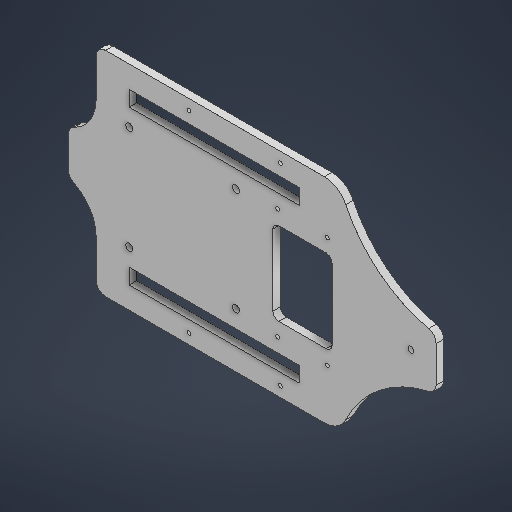
# Autodesk Inventor part: platform_deck
Saved by Autodesk Inventor 2026.1 (Build 301233020, 233B)
## iProperties
Created: 2026-01-28
Part Number: platform_deck
Material: Genérico
Document SubType Name: Modeling
Designer: i5
Density: 1 g/cm^3
Appearance: Valor por defecto
Author: i5
Autodesk Inventor part; units mm, degrees
ref_plane "YZ Plane" through (0, 0, 0) normal (1, 0, 0) x (0, 1, 0)
ref_plane "XZ Plane" through (0, 0, 0) normal (0, 1, 0) x (-1, 0, 0)
ref_plane "XY Plane" through (0, 0, 0) normal (0, 0, 1) x (1, 0, 0)
sketch "Boceto1" plane through (0, 0, 0) normal (0, 0, 1) x (1, 0, 0)
  line L0 (110.3805, 161.5) -> (194.7805, 161.5)
  line L1 (110.3805, 161.5) -> (194.7805, 161.5)
  line L2 (194.7805, 161.5) -> (194.7805, 148.5)
  line L3 (194.7805, 148.5) -> (110.3805, 148.5)
  line L4 (110.3805, 180) -> (216.0805, 180)
  line L5 (310.3805, 90) -> (310.3805, 105.2)
  arc A0 (310.3805, 105.2) -> (304.1178, 113.0091) centre (302.3805, 105.2) ccw
  arc A1 (234.1183, 168.6393) -> (216.0805, 180) centre (216.0805, 160) ccw
  arc A2 (234.1183, 168.6393) -> (304.1178, 113.0091) centre (326.3176, 212.7984) ccw
  line L6 (172.5805, 90) -> (172.5805, 120)
  line L7 (222.5805, 120) -> (222.5805, 90)
  circle A3 centre (289.0805, 90) radius 2.5
  circle A4 centre (141.4805, 133.75) radius 3
  line L8 (177.5805, 125) -> (197.5805, 125)
  arc A5 (177.5805, 125) -> (172.5805, 120) centre (177.5805, 120) ccw
  circle A6 centre (176.5805, 136.75) radius 1.65
  circle A7 centre (218.5805, 136.75) radius 1.65
  circle A8 centre (178.8805, 171.35) radius 1.65
  line L9 (197.5805, 125) -> (217.5805, 125)
  arc A9 (222.5805, 120) -> (217.5805, 125) centre (217.5805, 120) ccw
  line L10 (110.3805, 18.5) -> (194.7805, 18.5)
  line L11 (110.3805, 18.5) -> (194.7805, 18.5)
  line L12 (194.7805, 18.5) -> (194.7805, 31.5)
  line L13 (194.7805, 31.5) -> (110.3805, 31.5)
  line L14 (110.3805, 0) -> (216.0805, 0)
  line L15 (310.3805, 90) -> (310.3805, 74.8)
  arc A10 (304.1178, 66.9909) -> (310.3805, 74.8) centre (302.3805, 74.8) ccw
  arc A11 (216.0805, 0) -> (234.1183, 11.3607) centre (216.0805, 20) ccw
  arc A12 (304.1178, 66.9909) -> (234.1183, 11.3607) centre (326.3176, -32.7984) ccw
  line L16 (172.5805, 90) -> (172.5805, 60)
  line L17 (222.5805, 60) -> (222.5805, 90)
  circle A13 centre (289.0805, 90) radius 2.5
  circle A14 centre (141.4805, 46.25) radius 3
  line L18 (177.5805, 55) -> (197.5805, 55)
  arc A15 (172.5805, 60) -> (177.5805, 55) centre (177.5805, 60) ccw
  circle A16 centre (176.5805, 43.25) radius 1.65
  circle A17 centre (218.5805, 43.25) radius 1.65
  circle A18 centre (178.8805, 8.65) radius 1.65
  line L19 (197.5805, 55) -> (217.5805, 55)
  arc A19 (217.5805, 55) -> (222.5805, 60) centre (217.5805, 60) ccw
  line L20 (110.3805, 161.5) -> (51.3805, 161.5)
  line L21 (110.3805, 148.5) -> (51.3805, 148.5)
  line L22 (51.3805, 148.5) -> (51.3805, 161.5)
  line L23 (110.3805, 180) -> (31.3805, 180)
  line L24 (-0.0195, 90) -> (-0.0195, 103.12)
  arc A20 (4.5767, 110.3598) -> (-0.0195, 103.12) centre (7.9805, 103.12) ccw
  arc A21 (31.3805, 180) -> (23.3805, 172) centre (31.3805, 172) ccw
  arc A22 (4.5767, 110.3598) -> (23.3805, 139.9789) centre (-9.3489, 139.9789) ccw
  line L25 (23.3805, 139.9789) -> (23.3805, 172)
  circle A23 centre (101.7305, 171.35) radius 1.65
  circle A24 centre (51.3805, 133.9) radius 3
  line L26 (110.3805, 18.5) -> (51.3805, 18.5)
  line L27 (110.3805, 31.5) -> (51.3805, 31.5)
  line L28 (51.3805, 31.5) -> (51.3805, 18.5)
  line L29 (110.3805, 0) -> (31.3805, 0)
  line L30 (-0.0195, 90) -> (-0.0195, 76.88)
  arc A25 (-0.0195, 76.88) -> (4.5767, 69.6402) centre (7.9805, 76.88) ccw
  arc A26 (23.3805, 8) -> (31.3805, 0) centre (31.3805, 8) ccw
  arc A27 (23.3805, 40.0211) -> (4.5767, 69.6402) centre (-9.3489, 40.0211) ccw
  line L31 (23.3805, 40.0211) -> (23.3805, 8)
  circle A28 centre (101.7305, 8.65) radius 1.65
  circle A29 centre (51.3805, 46.1) radius 3
  point P0 (0, 0)
  constraints: 64 end point, 32 point on circle, 30 centre point
extrude "Extrusión1" add sketch "Boceto1" along normal blind 6.35
fillet "Empalme1" radius 0.01 44 edges at (25.7236, 177.6569, 6.35) (23.3805, 155.9894, 6.35) (18.2825, 122.437, 6.35) (1.2266, 107.4077, 6.35) (-0.0195, 96.56, 6.35) (-0.0195, 83.44, 6.35) (1.2266, 72.5923, 6.35) (18.2825, 57.563, 6.35) (23.3805, 24.0106, 6.35) (25.7236, 2.3431, 6.35) (70.8805, 0, 6.35) (163.2305, 0, 6.35) (226.7392, 3.0769, 6.35) (262.7136, 47.2345, 6.35) (308.6214, 69.7949, 6.35) (310.3805, 97.6, 6.35) (310.3805, 82.4, 6.35) (308.6214, 110.2051, 6.35) (262.7136, 132.7655, 6.35) (226.7392, 176.9231, 6.35) (70.8805, 180, 6.35) (163.2305, 180, 6.35) (25.7236, 177.6569, 0) (23.3805, 155.9894, 0) (18.2825, 122.437, 0) (1.2266, 107.4077, 0) (-0.0195, 96.56, 0) (-0.0195, 83.44, 0) (1.2266, 72.5923, 0) (18.2825, 57.563, 0) (23.3805, 24.0106, 0) (25.7236, 2.3431, 0) (70.8805, 0, 0) (163.2305, 0, 0) (226.7392, 3.0769, 0) (262.7136, 47.2345, 0) (308.6214, 69.7949, 0) (310.3805, 97.6, 0) (310.3805, 82.4, 0) (308.6214, 110.2051, 0) (262.7136, 132.7655, 0) (226.7392, 176.9231, 0) (70.8805, 180, 0) (163.2305, 180, 0)
